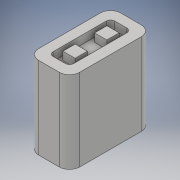
# Autodesk Inventor part: Automoblox Body
Saved by Autodesk Inventor 2018 (Build 220112000, 112)
## iProperties
Created: 2019-01-07
Part Number: Automoblox Body
Material: Generic
Document SubType Name: Modeling
Designer: 10043883
Density: 1 g/cm^3
Appearance: Default
Author: 10043883
Autodesk Inventor part; units mm, degrees
ref_plane "YZ Plane" through (0, 0, 0) normal (1, 0, 0) x (0, 1, 0)
ref_plane "XZ Plane" through (0, 0, 0) normal (0, 1, 0) x (-1, 0, 0)
ref_plane "XY Plane" through (0, 0, 0) normal (0, 0, 1) x (1, 0, 0)
sketch "Sketch2" plane through (0, 0, 0) normal (0, 1, 0) x (-1, 0, 0)
  line L0 (12.2483, 16.0201) -> (-0.4517, 16.0201)
  line L1 (-0.4517, 16.0201) -> (-0.4517, -9.3799)
  line L2 (-0.4517, -9.3799) -> (12.2483, -9.3799)
  line L3 (12.2483, -9.3799) -> (12.2483, 16.0201)
  point P0 (0, 0)
  dimension "d0" = 12.7
  dimension "d1" = 25.4
  constraints: 8 end point, 2 parallel, 1 horizontal, 1 perpendicular
  measures "d0" distance of L2.end L1.end
  measures "d1" distance of L1.end L0.end
extrude "Extrusion1" add sketch "Sketch2" along normal blind 25.4
fillet "Fillet1" radius 3.175 4 edges at (-12.2483, 12.7, -9.3799) (0.4517, 12.7, -9.3799) (-12.2483, 12.7, 16.0201) (0.4517, 12.7, 16.0201)
sketch "Sketch3" plane through (0, 0, 0) normal (0, -1, 0) x (1, 0, 0)
  line L0 (-2.8421, 12.9727) -> (-9.1921, 12.9727)
  line L1 (-9.1921, 12.9727) -> (-9.1921, -6.0773)
  line L2 (-9.1921, -6.0773) -> (-2.8421, -6.0773)
  line L3 (-2.8421, -6.0773) -> (-2.8421, 12.9727)
  point P0 (0, 0)
  dimension "d5" = 6.35
  dimension "d6" = 19.05
  constraints: 8 end point, 2 parallel, 1 horizontal, 1 perpendicular
  measures "d5" distance of L2.end L1.end
  measures "d6" distance of L1.end L0.end
extrude "Extrusion2" cut sketch "Sketch3" against normal blind 2.54
fillet "Fillet2" radius 1.524 4 edges at (-9.1921, 1.27, 12.9727) (-9.1921, 1.27, -6.0773) (-2.8421, 1.27, 12.9727) (-2.8421, 1.27, -6.0773)
sketch "Sketch4" plane through (0.0246, 25.4, 6.6784) normal (0, 1, 0) x (1, 0, 0)
  line L0 (-2.8421, 12.9727) -> (-9.1921, 12.9727)
  line L1 (-9.1921, 12.9727) -> (-9.1921, -6.0773)
  line L2 (-9.1921, -6.0773) -> (-2.8421, -6.0773)
  line L3 (-2.8421, -6.0773) -> (-2.8421, 12.9727)
  point P0 (0, 0)
  dimension "d10" = 6.35
  dimension "d11" = 19.05
  constraints: 8 end point, 2 parallel, 1 horizontal, 1 perpendicular
  measures "d10" distance of L2.end L1.end
  measures "d11" distance of L1.end L0.end
extrude "Extrusion3" cut sketch "Sketch4" against normal blind 2.54
fillet "Fillet3" radius 1.27 4 edges at (-9.1674, 24.13, -6.2944) (-2.8174, 24.13, -6.2944) (-9.1674, 24.13, 12.7556) (-2.8174, 24.13, 12.7556)
sketch "Sketch6" plane through (0.0246, 22.86, 6.6784) normal (0, 1, 0) x (1, 0, 0)
  line L0 (-7.8199, -3.1416) -> (-4.0099, -3.1416)
  line L1 (-4.0099, -3.1416) -> (-4.0099, 0.6684)
  line L2 (-4.0099, 0.6684) -> (-7.8199, 0.6684)
  line L3 (-7.8199, 0.6684) -> (-7.8199, -3.1416)
  line L4 (-7.8199, 6.6784) -> (-4.0099, 6.6784)
  line L5 (-4.0099, 6.6784) -> (-4.0099, 10.4884)
  line L6 (-4.0099, 10.4884) -> (-7.8199, 10.4884)
  line L7 (-7.8199, 10.4884) -> (-7.8199, 6.6784)
  point P0 (-0.0246, 6.6784)
  dimension "d16" = 3.81
  dimension "d17" = 3.81
  dimension "d18" = 3.81
  dimension "d19" = 3.81
  constraints: 16 end point, 4 parallel, 2 horizontal, 2 perpendicular
  measures "d16" distance of L2.end L1.end
  measures "d17" distance of L1.end L0.end
  measures "d18" distance of L6.end L5.end
  measures "d19" distance of L5.end L4.end
extrude "Extrusion4" add sketch "Sketch6" along normal blind 2.54
sketch "Sketch7" plane through (-0.3446, 2.54, -0.3565) normal (0, -1, 0) x (1, 0, 0)
  line L0 (-7.8199, -3.1416) -> (-4.0099, -3.1416)
  line L1 (-4.0099, -3.1416) -> (-4.0099, 0.6684)
  line L2 (-4.0099, 0.6684) -> (-7.8199, 0.6684)
  line L3 (-7.8199, 0.6684) -> (-7.8199, -3.1416)
  line L4 (-7.8199, 6.6784) -> (-4.0099, 6.6784)
  line L5 (-4.0099, 6.6784) -> (-4.0099, 10.4884)
  line L6 (-4.0099, 10.4884) -> (-7.8199, 10.4884)
  line L7 (-7.8199, 10.4884) -> (-7.8199, 6.6784)
  point P0 (-0.0246, 6.6784)
  dimension "d24" = 3.81
  dimension "d25" = 3.81
  dimension "d22" = 3.81
  dimension "d23" = 3.81
  constraints: 16 end point, 4 parallel, 2 horizontal, 2 perpendicular
  measures "d24" distance of L2.end L1.end
  measures "d25" distance of L1.end L0.end
  measures "d22" distance of L6.end L5.end
  measures "d23" distance of L5.end L4.end
extrude "Extrusion5" add sketch "Sketch7" along normal blind 2.54
sketch "Sketch8" plane through (-12.2483, 0, -6.2049) normal (-1, 0, 0) x (0, 0, 1)
  point P0 (6.2049, 0)
sketch "Sketch9" plane through (-12.2483, 0, -6.2049) normal (-1, 0, 0) x (0, 0, 1)
  point P0 (6.2049, 0)
sketch "Sketch10" plane through (-12.2483, 0, -6.2049) normal (-1, 0, 0) x (0, 0, 1)
  line L0 (19.05, 25.4) -> (19.05, 0) projected
  line L1 (0, 0) -> (0, 25.4) projected
  line L2 (19.05, 18.7302) -> (0, 18.7302)
  line L3 (0, 18.7302) -> (0, 6.0302)
  line L4 (0, 6.0302) -> (19.05, 6.0302)
  line L5 (19.05, 6.0302) -> (19.05, 18.7302)
  point P0 (6.2049, 0)
  dimension "d29" = 12.7
  constraints: 8 end point, 2 parallel, 2 point on line, 1 horizontal, 1 perpendicular
  measures "d29" distance of L3.end L2.end
extrude "Extrusion6" cut sketch "Sketch10" against normal blind 10.16
fillet "Fillet4" radius 1.27 4 edges at (-7.1683, 18.7302, 12.8451) (-7.1683, 6.0302, 12.8451) (-7.1683, 18.7302, -6.2049) (-7.1683, 6.0302, -6.2049)
body "Solid1"
